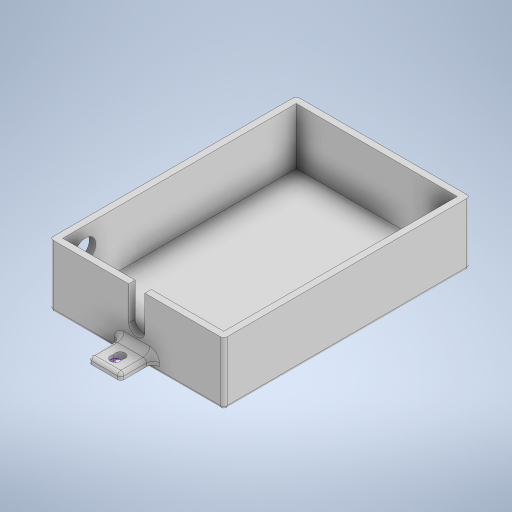
# Autodesk Inventor part: Golf Cart Mainboard Box
Saved by Autodesk Inventor 2024 (Build 280153000, 153)
## iProperties
Created: 2023-08-07
Part Number: Golf Cart Mainboard Box
Material: Generic
Document SubType Name: Modeling
Designer: techn
Density: 1 g/cm^3
Appearance: Default
Author: techn
## iProperties of the stored document Golf Cart Mainboard Box_3DPrint.ipt
Created: 2023-08-07
Part Number: Golf Cart Mainboard Box_3DPrint
Material: Generic
Document SubType Name: Modeling
Designer: techn
Density: 1 g/cm^3
Appearance: Default
Author: techn
Autodesk Inventor part; units mm, degrees
ref_plane "YZ Plane" through (0, 0, 0) normal (1, 0, 0) x (0, 1, 0)
ref_plane "XZ Plane" through (0, 0, 0) normal (0, 1, 0) x (-1, 0, 0)
ref_plane "XY Plane" through (0, 0, 0) normal (0, 0, 1) x (1, 0, 0)
sketch "Sketch2" plane through (0, 0, 0) normal (0, 1, 0) x (-1, 0, 0)
  line L0 (0, 0) -> (-108, 0)
  line L1 (-108, 0) -> (-108, 153)
  line L2 (-108, 153) -> (0, 153)
  line L3 (0, 153) -> (0, 0)
  line L4 (-44, 153) -> (-64, 153)
  line L5 (-64, 153) -> (-64, 168)
  line L6 (-64, 168) -> (-44, 168)
  line L7 (-44, 168) -> (-44, 153)
  line L8 (-44, 0) -> (-64, 0)
  line L9 (-64, 0) -> (-64, -15)
  line L10 (-64, -15) -> (-44, -15)
  line L11 (-44, -15) -> (-44, 0)
  dimension "d0" = 108
  dimension "d1" = 153
  dimension "d2" = 20
  dimension "d3" = 15
  dimension "d4" = 20
  dimension "d5" = 15
  constraints: 24 end point, 6 parallel, 3 horizontal, 3 perpendicular, 2 point on line
  measures "d0" distance of L1.end L2.end
  measures "d1" distance of L0.end L1.end
  measures "d2" distance of L5.end L6.end
  measures "d3" distance of L4.end L5.end
  measures "d4" distance of L10.end L9.end
  measures "d5" distance of L9.end L8.end
extrude "Extrusion1" add sketch "Sketch2" along normal blind 4
sketch "Sketch3" plane through (0, 4, 0) normal (0, 1, 0) x (1, 0, 0)
  line L0 (44, 0) -> (0, 0) projected
  line L1 (0, 0) -> (4, 0)
  line L2 (4, 0) -> (4, -4)
  line L3 (4, -4) -> (0, -4)
  line L4 (0, -4) -> (0, 0)
  line L5 (4, -4) -> (104, -4)
  line L6 (104, -4) -> (104, -149)
  line L7 (104, -149) -> (4, -149)
  line L8 (4, -149) -> (4, -4)
  line L9 (108, -153) -> (108, 0) projected
  line L10 (108, -153) -> (0, -153)
  line L11 (0, -153) -> (0, 0)
  line L12 (0, 0) -> (108, 0)
  line L13 (108, 0) -> (108, -153)
  line L14 (64, 0) -> (64, 15) projected
  line L15 (44, 15) -> (44, 0) projected
  line L16 (64, 15) -> (44, 15)
  line L17 (44, 15) -> (44, 0)
  line L18 (44, 0) -> (64, 0)
  line L19 (64, 0) -> (64, 15)
  line L20 (44, -168) -> (64, -168) projected
  line L21 (64, -153) -> (44, -153)
  line L22 (44, -153) -> (44, -168)
  line L23 (44, -168) -> (64, -168)
  line L24 (64, -168) -> (64, -153)
  dimension "d8" = 4
  dimension "d9" = 4
  dimension "d10" = 100
  dimension "d11" = 145
  constraints: 40 end point, 10 parallel, 5 horizontal, 5 perpendicular, 2 point on line
  measures "d8" distance of L2.end L3.end
  measures "d9" distance of L1.end L2.end
  measures "d10" distance of L6.end L7.end
  measures "d11" distance of L5.end L6.end
extrude "Extrusion2" add sketch "Sketch3" along normal blind 35 contours L12 L9 L10 L11 L3 L2 L0 | L2 L3 L4 L0
sketch "Sketch4" plane through (0, 4, 0) normal (0, 1, 0) x (1, 0, 0)
  line L0 (44, -168) -> (64, -168) projected
  line L1 (44, -168) -> (54, -168)
  line L2 (54, -168) -> (54, -160.5)
  line L3 (54, -160.5) -> (44, -160.5)
  line L4 (44, -160.5) -> (44, -168)
  circle A0 centre (54, -160.5) radius 2.75
  circle A1 centre (54, 7.5) radius 2.75
  point P0 (0, 0)
  dimension "d14" = 7.5
  dimension "d15" = 5.5
  dimension "d16" = 5.5
  constraints: 8 end point, 2 centre point, 2 parallel, 1 coincident, 1 horizontal, 1 perpendicular
  measures "d14" distance of L2.end L1.end
  measures "d15" diameter of A0
  measures "d16" diameter of A1
extrude "Extrusion3" cut sketch "Sketch4" against normal blind 35 contours A0 L3 L2 | L2 L3 A0 | A1
sketch "Sketch5" plane through (0, 4, 0) normal (0, 1, 0) x (1, 0, 0)
  line L0 (44, -153) -> (44, -168) projected
  line L1 (64, -168) -> (64, -153) projected
  line L2 (44, -153) -> (64, -153)
  line L3 (64, -153) -> (64, -168)
  line L4 (64, -168) -> (44, -168)
  line L5 (44, -168) -> (44, -153)
  circle A0 centre (54, -160.5) radius 2.75 projected
  circle A1 centre (54, -160.5) radius 2.75
  point P0 (0, 0)
  constraints: 8 end point, 2 parallel, 1 centre point, 1 coincident, 1 horizontal, 1 perpendicular
extrude "Extrusion4" add sketch "Sketch5" along normal blind 3
sketch "Sketch6" plane through (0, 0, 0) normal (0, -1, 0) x (1, 0, 0)
  line L0 (44, 153) -> (44, 168) projected
  line L1 (44, 153) -> (64, 153) projected
  line L2 (44, 168) -> (64, 168)
  line L3 (64, 168) -> (64, 153)
  line L4 (64, 153) -> (44, 153)
  line L5 (44, 153) -> (44, 168)
  circle A0 centre (54, 160.5) radius 2.75 projected
  circle A1 centre (54, 160.5) radius 2.75
  point P0 (0, 0)
  constraints: 8 end point, 2 parallel, 1 centre point, 1 coincident, 1 horizontal, 1 perpendicular
extrude "Extrusion5" cut sketch "Sketch6" against normal blind 3
sketch "Sketch7" plane through (0, 0, 0) normal (-1, 0, 0) x (0, 0, 1)
  line L0 (0, 39) -> (153, 39) projected
  line L1 (153, 39) -> (128, 39)
  line L2 (128, 39) -> (128, 26)
  line L3 (128, 26) -> (153, 26)
  line L4 (153, 26) -> (153, 39)
  circle A0 centre (128, 26) radius 6
  point P0 (0, 0)
  dimension "d23" = 25
  dimension "d24" = 13
  dimension "d25" = 12
  constraints: 8 end point, 2 parallel, 1 centre point, 1 coincident, 1 horizontal, 1 perpendicular
  measures "d23" distance of L3.end L2.end
  measures "d24" distance of L2.end L1.end
  measures "d25" diameter of A0
extrude "Extrusion6" cut sketch "Sketch7" against normal blind 4 contours A0 L3 L2 | L2 L3 A0
sketch "Sketch8" plane through (0, 0, 153) normal (0, 0, 1) x (1, 0, 0)
  line L0 (0, 0) -> (0, 39) projected
  line L1 (0, 39) -> (54, 39)
  line L2 (54, 39) -> (54, 14)
  line L3 (54, 14) -> (0, 14)
  line L4 (0, 14) -> (0, 39)
  circle A0 centre (54, 18) radius 4
  line L5 (108, 39) -> (0, 39) projected
  line L6 (50, 18) -> (58, 18)
  line L7 (58, 18) -> (58, 39)
  line L8 (58, 39) -> (50, 39)
  line L9 (50, 39) -> (50, 18)
  dimension "d28" = 54
  dimension "d29" = 25
  constraints: 16 end point, 4 parallel, 2 horizontal, 2 perpendicular, 2 point on circle, 2 point on line, 1 centre point
  measures "d28" distance of L2.end L3.end
  measures "d29" distance of L1.end L2.end
extrude "Extrusion7" cut sketch "Sketch8" against normal blind 50 contours A0 L6 L2 | L2 L6 A0 | L1 L2 A0 L9 | L6 A0 L2 | L2 A0 L6 | A0 L2 L5 L7
sketch "Sketch9" plane through (0, 3, 0) normal (0, -1, 0) x (1, 0, 0)
  point P0 (0, 0)
sketch "Sketch10" plane through (0, 3, 0) normal (0, -1, 0) x (1, 0, 0)
  line L0 (44, 153) -> (44, 168) projected
  line L1 (44, 168) -> (64, 168)
  line L2 (64, 168) -> (64, 153)
  line L3 (64, 153) -> (44, 153)
  line L4 (44, 153) -> (44, 168)
  circle A0 centre (54, 160.5) radius 2.75 projected
  circle A1 centre (54, 160.5) radius 2.75
  point P0 (0, 0)
  constraints: 8 end point, 2 parallel, 1 centre point, 1 coincident, 1 horizontal, 1 perpendicular
extrude "Extrusion8" cut sketch "Sketch10" against normal blind 3
sketch "Sketch11" plane through (0, 7, 0) normal (0, 1, 0) x (1, 0, 0)
  line L0 (44, -168) -> (64, -168) projected
  line L1 (44, -153) -> (64, -153) projected
  line L2 (44, -168) -> (64, -168)
  line L3 (64, -168) -> (64, -153)
  line L4 (64, -153) -> (44, -153)
  line L5 (44, -153) -> (44, -168)
  circle A0 centre (54, -160.5) radius 2.75
  point P0 (0, 0)
  constraints: 8 end point, 2 parallel, 1 centre point, 1 horizontal, 1 perpendicular
extrude "Extrusion9" add sketch "Sketch11" along normal blind 3
sketch "Sketch12" plane through (44, 6, 168) normal (0, 0, 1) x (1, 0, 0)
  line L0 (20, 0) -> (20, 4) projected
  line L1 (0, 0) -> (20, 0)
  line L2 (20, 0) -> (20, 4)
  line L3 (20, 4) -> (0, 4)
  line L4 (0, 4) -> (0, 0)
  point P0 (-44, -6)
  constraints: 8 end point, 2 parallel, 1 horizontal, 1 perpendicular
extrude "Extrusion10" add sketch "Sketch12" along normal blind 5
sketch "Sketch13" plane through (0, 10, 0) normal (0, 1, 0) x (1, 0, 0)
  circle A0 centre (54, -160.5) radius 2.75 projected
  circle A1 centre (54, -160.5) radius 2.75
  point P0 (0, 0)
  constraints: 1 centre point, 1 coincident
extrude "Extrusion11" add sketch "Sketch13" against normal blind 4
sketch "Sketch14" plane through (0, 10, 0) normal (0, 1, 0) x (1, 0, 0)
  point P0 (0, 0)
sketch "Sketch15" plane through (0, 10, 0) normal (0, 1, 0) x (1, 0, 0)
  circle A0 centre (54, -166.3159) radius 3
  point P0 (0, 0)
  dimension "d42" = 6
  constraints: 1 centre point
  measures "d42" diameter of A0
extrude "Extrusion12" cut sketch "Sketch15" against normal blind 4
sketch "Sketch16" plane through (0, 4, 0) normal (0, 1, 0) x (1, 0, 0)
  circle A0 centre (54, 7.5) radius 2.75 projected
  circle A1 centre (54, 7.5) radius 3
  point P0 (0, 0)
  dimension "d45" = 6
  constraints: 1 centre point, 1 coincident
  measures "d45" diameter of A1
extrude "Extrusion13" cut sketch "Sketch16" against normal blind 4 contours A0 | A1
sketch "Sketch17" plane through (0, 0, 0) normal (-1, 0, 0) x (0, 0, 1)
  circle A0 centre (128, 26) radius 6 projected
  circle A1 centre (128, 26) radius 6.25
  circle A2 centre (128, 26) radius 6.75
  point P0 (0, 0)
  dimension "d48" = 12.5
  dimension "d49" = 13.5
  constraints: 2 centre point, 2 coincident
  measures "d48" diameter of A1
  measures "d49" diameter of A2
extrude "Extrusion14" cut sketch "Sketch17" against normal blind 4 contours A0 | A1 | A2
sketch "Sketch18" plane through (0, 0, 153) normal (0, 0, 1) x (1, 0, 0)
  arc A0 (50, 18) -> (58, 18) centre (54, 18) ccw projected
  circle A1 centre (54, 18) radius 5
  line L0 (49, 18) -> (49, 39)
  line L1 (0, 39) -> (50, 39) projected
  line L2 (59, 18) -> (59, 39)
  line L3 (58, 39) -> (108, 39) projected
  line L4 (49, 39) -> (59, 39)
  point P0 (0, 0)
  dimension "d52" = 10
  constraints: 6 end point, 2 point on circle, 2 point on line, 1 centre point, 1 coincident, 1 parallel, 1 perpendicular, 1 vertical
  measures "d52" diameter of A1
extrude "Extrusion15" cut sketch "Sketch18" against normal blind 4
sketch "Sketch19" plane through (0, 6, 0) normal (0, -1, 0) x (1, 0, 0)
  line L0 (44, 173) -> (64, 173) projected
  line L1 (44, 173) -> (64, 173)
  line L2 (64, 173) -> (64, 153)
  line L3 (64, 153) -> (44, 153)
  line L4 (44, 153) -> (44, 173)
  point P0 (0, 0)
  constraints: 8 end point, 2 parallel, 1 horizontal, 1 perpendicular
extrude "Extrusion16" add sketch "Sketch19" along normal blind 2
sketch "Sketch20" plane through (0, 10, 0) normal (0, 1, 0) x (1, 0, 0)
  line L0 (64, -153) -> (64, -173) projected
  line L1 (44, -153) -> (64, -153)
  line L2 (64, -153) -> (64, -173)
  line L3 (64, -173) -> (44, -173)
  line L4 (44, -173) -> (44, -153)
  point P0 (0, 0)
  constraints: 8 end point, 2 parallel, 1 horizontal, 1 perpendicular
extrude "Extrusion17" cut sketch "Sketch20" against normal blind 2
sketch "Sketch21" plane through (54, 6, 166.3159) normal (0, 1, 0) x (1, 0, 0)
  circle A0 centre (0, 0) radius 3
  point P0 (-54, 166.3159)
  constraints: 1 centre point
sketch "Sketch22" plane through (0, 8, 0) normal (0, 1, 0) x (1, 0, 0)
  circle A0 centre (54, -166.3159) radius 3 projected
  circle A1 centre (54, -163.3159) radius 3
  point P0 (0, 0)
  point P1 (56.5981, -164.8159)
  point P2 (51.4019, -164.8159)
  constraints: 1 centre point, 2 other
extrude "Extrusion18" cut sketch "Sketch22" against normal blind 5 contours A0 A1 picked at (53.8493, -161.3379)
sketch "Sketch23" plane through (0, 6, 0) normal (0, 1, 0) x (1, 0, 0)
  point P0 (0, 0)
sketch "Sketch24" plane through (0, 6, 0) normal (0, 1, 0) x (1, 0, 0)
  arc A0 (56.5981, -164.8159) -> (51.4019, -164.8159) centre (54, -166.3159) ccw projected
  circle A1 centre (54, -166.3159) radius 3
  point P0 (0, 0)
  point P1 (51.4019, -164.8159)
  point P2 (56.5981, -164.8159)
  constraints: 1 centre point, 1 coincident
extrude "Extrusion19" cut sketch "Sketch24" against normal blind 5
sketch "Sketch25" plane through (0, 0, 0) normal (-1, 0, 0) x (0, 0, 1)
  circle A0 centre (128, 26) radius 6.75 projected
  circle A1 centre (128, 26) radius 6.75
  point P0 (0, 0)
  constraints: 1 centre point, 1 coincident
extrude "Extrusion20" add sketch "Sketch25" against normal blind 4
sketch "Sketch26" plane through (0, 0, 0) normal (-1, 0, 0) x (0, 0, 1)
  circle A0 centre (134.9231, 29.4176) radius 6.375
  circle A1 centre (134.9231, 25.7949) radius 6.375
  point P0 (0, 0)
  dimension "d65" = 12.75
  dimension "d66" = 12.75
  constraints: 2 centre point
  measures "d65" diameter of A0
  measures "d66" diameter of A1
extrude "Extrusion21" cut sketch "Sketch26" against normal blind 4 contours A1 A0 | A0 A1 picked at (134.6759, 26.0995) picked at (134.5849, 20.6747)
fillet "Fillet4" radius 4 1 edges at (54, 4, 0)
fillet "Fillet5" radius 2 21 edges at (0, 19.5, 0) (0, 0, 76.5) (22, 0, 0) (44, 5.1716, -1.1716) (44, 4, -9.5) (54, 4, -15) (64, 5.1716, -1.1716) (64, 4, -9.5) (64, 2, -15) (44, 2, -15) (108, 19.5, 0) (86, 0, 0) (108, 0, 76.5) (108, 19.5, 153) (54, 0, 153) (0, 19.5, 153) (44, 8, 163) (44, 6, 173) (54, 8, 173) (64, 8, 163) (64, 6, 173)
fillet "Fillet6" radius 4 5 edges at (63.4142, 7.4142, 153) (64, 5, 153) (44.5858, 7.4142, 153) (44, 5, 153) (54, 8, 153)
body "Solid1"
